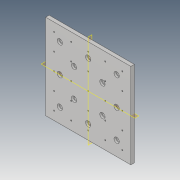
# Autodesk Inventor part: J010183
Saved by Autodesk Inventor 2020.4 (Build 244396000, 396)
## iProperties
Created: 2020-08-24
Part Number: J010183
Material: ALUMINUM, 6061-T651
Document SubType Name: Modeling
Designer: sawtelles
Density: 2.7 g/cm^3
Appearance: Metal-AL-6061 (Machined)
Project: COMMON
Description: RGB2THOR HEATSINK CENTERED
Vendor: HHMI: JRC - JET
ALTERED ITEM PART NUMBER: N/A
ALTERED ITEM VENDOR: N/A
ALTERED ITEM DESCRIPTION: N/A
DESIGN DEPARTMENT: HHMI: JRC - ID&F
LAB/DEPT: COMMON
REQUESTING SCIENTIST: COMMON
SPECIAL FINISH: ANODIZE PER MIL-A-8625F, TYPE II, CLASS 2 (BLACK)
SURFACE ROUGHNESS: 63 Ra
PART NUMBER - LEGACY: J010181
Author: sawtelles
Revision Number: -
Autodesk Inventor part; units mm, degrees
ref_plane "YZ Plane" through (0, 0, 0) normal (1, 0, 0) x (0, 1, 0)
ref_plane "XZ Plane" through (0, 0, 0) normal (0, 1, 0) x (-1, 0, 0)
ref_plane "XY Plane" through (0, 0, 0) normal (0, 0, 1) x (1, 0, 0)
sketch "Sketch1" plane through (0, 0, 0) normal (0, 0, 1) x (1, 0, 0)
  line L0 (0, 0) -> (152.4, 0)
  line L1 (152.4, 0) -> (152.4, 152.4)
  line L2 (152.4, 152.4) -> (0, 152.4)
  line L3 (0, 152.4) -> (0, 0)
  dimension "d0" = 152.4
  dimension "d1" = 152.4
  constraints: 8 end point, 2 parallel, 1 horizontal, 1 perpendicular
  measures "d0" distance of L2.end L1.end
  measures "d1" distance of L1.end L0.end
extrude "Extrusion1" add sketch "Sketch1" along normal blind 6.35
sketch "Sketch2" plane through (0, 0, 6.35) normal (0, 0, 1) x (1, 0, 0)
  point P0 (0, 0)
  point P1 (15.24, 15.24)
  point P2 (45.72, 15.24)
  point P3 (76.2, 15.24)
  point P4 (106.68, 15.24)
  point P5 (137.16, 15.24)
  point P6 (15.24, 45.72)
  point P7 (45.72, 45.72)
  point P8 (76.2, 45.72)
  point P9 (106.68, 45.72)
  point P10 (137.16, 45.72)
  point P11 (137.16, 76.2)
  point P12 (106.68, 76.2)
  point P13 (76.2, 76.2)
  point P14 (45.72, 76.2)
  point P15 (15.24, 76.2)
  point P16 (15.24, 106.68)
  point P17 (45.72, 106.68)
  point P18 (76.2, 106.68)
  point P19 (106.68, 106.68)
  point P20 (137.16, 106.68)
  point P21 (137.16, 137.16)
  point P22 (106.68, 137.16)
  point P23 (76.2, 137.16)
  point P24 (45.72, 137.16)
  point P25 (15.24, 137.16)
hole "Hole1" at (15.24, 15.24, 6.35) at (45.72, 15.24, 6.35) at (76.2, 15.24, 6.35) at (106.68, 15.24, 6.35) at (137.16, 15.24, 6.35) at (15.24, 45.72, 6.35) at (45.72, 45.72, 6.35) at (76.2, 45.72, 6.35) at (106.68, 45.72, 6.35) at (137.16, 45.72, 6.35) at (137.16, 76.2, 6.35) at (106.68, 76.2, 6.35) at (76.2, 76.2, 6.35) at (45.72, 76.2, 6.35) at (15.24, 76.2, 6.35) at (15.24, 106.68, 6.35) at (45.72, 106.68, 6.35) at (76.2, 106.68, 6.35) at (106.68, 106.68, 6.35) at (137.16, 106.68, 6.35) at (137.16, 137.16, 6.35) at (106.68, 137.16, 6.35) at (76.2, 137.16, 6.35) at (45.72, 137.16, 6.35) at (15.24, 137.16, 6.35) direction (0, 0, -1) diameter 2.159 end through all
sketch "Sketch3" plane through (0, 0, 6.35) normal (0, 0, 1) x (1, 0, 0)
  line L0 (0, 0) -> (152.4, 0) projected
  line L1 (0, 152.4) -> (0, 0) projected
  point P0 (76.2, 25.4)
  point P1 (127, 25.4)
  point P2 (127, 127)
  point P3 (25.4, 25.8124)
  point P4 (50.8, 50.8)
  point P5 (127, 76.2)
  point P6 (101.6, 50.8)
  point P7 (50.8, 101.6)
  point P8 (25.4, 76.2)
  point P9 (25.4, 127)
  point P10 (76.2, 127)
  point P11 (101.6, 101.6)
  dimension "d19" = 25.4
  dimension "d21" = 25.4
  dimension "d23" = 25.4
  dimension "d25" = 76.2
  dimension "d27" = 127
  dimension "d28" = 76.2
  dimension "d30" = 127
  dimension "d33" = 50.8
  dimension "d38" = 50.8
  dimension "d40" = 101.6
  dimension "d42" = 50.8
  dimension "d43" = 50.8
  dimension "d46" = 25.4
  dimension "d48" = 25.4
  dimension "d55" = 50.8
  dimension "d56" = 101.6
  measures "d19" distance from line of L0 point (76.2, 25.4)
  measures "d21" distance from line of L0 point (127, 25.4)
  measures "d23" distance from line of L1 point (25.4, 25.812)
  measures "d25" distance from line of L1 point (76.2, 25.4)
  measures "d27" distance from line of L1 point (127, 25.4)
  measures "d28" distance from line of L0 point (25.4, 76.2)
  measures "d30" distance from line of L0 point (25.4, 127)
  measures "d33" distance of point (101.6, 50.8) point (50.8, 50.8)
  measures "d38" distance of point (101.6, 101.6) point (50.8, 101.6)
  measures "d40" distance of point (127, 76.2) point (25.4, 76.2)
  measures "d42" distance of point (50.8, 50.8) point (50.8, 101.6)
  measures "d43" distance of point (101.6, 50.8) point (101.6, 101.6)
  measures "d46" distance from line of L1 point (25.4, 76.2)
  measures "d48" distance from line of L1 point (25.4, 127)
  measures "d55" distance of point (76.2, 127) point (25.4, 127)
  measures "d56" distance of point (76.2, 25.4) point (76.2, 127)
hole "Hole2" at (76.2, 25.4, 6.35) at (127, 25.4, 6.35) at (127, 127, 6.35) at (25.4, 25.8124, 6.35) at (50.8, 50.8, 6.35) at (127, 76.2, 6.35) at (101.6, 50.8, 6.35) at (50.8, 101.6, 6.35) at (25.4, 76.2, 6.35) at (25.4, 127, 6.35) at (76.2, 127, 6.35) at (101.6, 101.6, 6.35) direction (0, 0, -1) diameter 6.35 end through all counterbore diameter 9.525 counterbore depth 3.302
ref_plane "Work Plane1" through (0, 76.2, 0) normal (0, 1, 0) x (1, 0, 0)
ref_plane "Work Plane2" through (76.2, 0, 0) normal (1, 0, 0) x (0, 0, -1)
body "Solid1"
